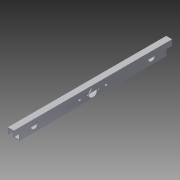
# Autodesk Inventor part: chassis side rail
Saved by Autodesk Inventor 2014 SP1 (Build 180222100, 222)
## iProperties
Created: 2014-01-04
Part Number: chassis side rail
Material: Aluminum 6061
Document SubType Name: Modeling
Designer: Arpan
Density: 2.71 g/cm^3
Appearance: Aluminum - Flat
Author: Arpan
Autodesk Inventor part; units mm, degrees
ref_plane "YZ Plane" through (0, 0, 0) normal (1, 0, 0) x (0, 1, 0)
ref_plane "XZ Plane" through (0, 0, 0) normal (0, 1, 0) x (-1, 0, 0)
ref_plane "XY Plane" through (0, 0, 0) normal (0, 0, 1) x (1, 0, 0)
sketch "Sketch1" plane through (0, 0, 0) normal (0, 0, 1) x (1, 0, 0)
  line L0 (0, 0) -> (-25.4, 0)
  line L1 (-25.4, 0) -> (-25.4, 50.8)
  line L2 (-25.4, 50.8) -> (0, 50.8)
  line L3 (0, 50.8) -> (0, 0)
  line L4 (-3.175, 47.625) -> (-22.225, 47.625)
  line L5 (-22.225, 47.625) -> (-22.225, 3.175)
  line L6 (-22.225, 3.175) -> (-3.175, 3.175)
  line L7 (-3.175, 3.175) -> (-3.175, 47.625)
  dimension "d0" = 25.4
  dimension "d1" = 50.8
  dimension "d2" = 3.175
  constraints: 16 end point, 4 parallel, 2 perpendicular, 1 horizontal, 3 other
  measures "d0" distance of L1.end L2.end
  measures "d1" distance of L2.end L0.start
  measures "d2" distance between parallel lines of L2 L4
extrude "Extrusion1" add sketch "Sketch1" along normal blind 685.8
sketch "Sketch2" plane through (0, 0, 0) normal (1, 0, 0) x (0, 0, -1)
  line L0 (0, 50.8) -> (0, 0) projected
  line L1 (-685.8, 0) -> (-685.8, 50.8) projected
  line L2 (0, 0) -> (-685.8, 0) projected
  line L3 (-685.8, 0) -> (-685.8, 25.4)
  line L4 (-685.8, 25.4) -> (-660.4, 25.4)
  line L5 (-660.4, 25.4) -> (-660.4, 0)
  line L6 (0, 25.4) -> (-25.4, 25.4)
  line L7 (-25.4, 25.4) -> (-25.4, 0)
  dimension "d5" = 25.4
  dimension "d6" = 25.4
  dimension "d7" = 25.4
  constraints: 10 end point, 4 perpendicular, 2 midpoint, 2 point on line
  measures "d5" distance of L1.start L3.end
  measures "d6" distance of L3.end L4.end
  measures "d7" distance of L6.start L6.end
extrude "Extrusion2" cut sketch "Sketch2" against normal blind 685.8
sketch "Sketch3" plane through (-25.4, 50.8, 0) normal (-1, 0, 0) x (0, 0, 1)
  line L0 (25.4, -50.8) -> (660.4, -50.8) projected
  line L1 (25.4, -50.8) -> (88.9, -50.8)
  line L2 (88.9, -50.8) -> (88.9, -23.8125)
  circle A0 centre (88.9, -23.8125) radius 14.2875
  line L3 (660.4, -50.8) -> (596.9, -50.8)
  line L4 (596.9, -50.8) -> (596.9, -23.8125)
  circle A1 centre (596.9, -23.8125) radius 14.2875
  line L5 (88.9, -50.8) -> (342.9, -50.8)
  line L6 (342.9, -50.8) -> (342.9, -23.8125)
  line L7 (342.9, -23.8125) -> (342.9, -26.9875)
  circle A2 centre (342.9, -26.9875) radius 19.05
  point P0 (0, -50.8)
  dimension "d10" = 63.5
  dimension "d11" = 26.9875
  dimension "d12" = 28.575
  dimension "d13" = 63.5
  dimension "d14" = 28.575
  dimension "d16" = 3.175
  dimension "d18" = 38.1
  constraints: 14 end point, 3 centre point, 3 coincident, 3 perpendicular, 3 point on line, 2 horizontal alignment, 1 midpoint
  measures "d10" distance of L0.start L1.end
  measures "d11" distance of L1.end L2.end
  measures "d12" diameter of A0
  measures "d13" distance of L0.end L3.end
  measures "d14" diameter of A1
  measures "d16" distance of L6.end L7.end
  measures "d18" diameter of A2
extrude "Extrusion3" cut sketch "Sketch3" against normal blind 685.8
sketch "Sketch4" plane through (-25.4, 50.8, 0) normal (-1, 0, 0) x (0, 0, 1)
  circle A0 centre (342.9, -26.9875) radius 19.05 projected
  line L0 (0, -25.4) -> (0, 0) projected
  line L1 (342.9, -26.9875) -> (319.0748, -26.9875)
  circle A1 centre (319.0748, -26.9875) radius 2.54
  line L2 (342.9, -26.9875) -> (366.7252, -26.9875)
  circle A2 centre (366.7252, -26.9875) radius 2.54
  line L3 (342.9, -26.9875) -> (285.75, -26.9875)
  line L4 (342.9, -26.9875) -> (400.05, -26.9875)
  circle A3 centre (285.75, -26.9875) radius 5.08
  circle A4 centre (400.05, -26.9875) radius 5.08
  point P0 (0, -50.8)
  dimension "d21" = 23.8252
  dimension "d22" = 5.08
  dimension "d23" = 23.8252
  dimension "d24" = 5.08
  dimension "d25" = 57.15
  dimension "d26" = 57.15
  dimension "d27" = 10.16
  constraints: 8 end point, 4 centre point, 4 coincident, 3 collinear, 1 perpendicular
  measures "d21" distance of L1.start L1.end
  measures "d22" diameter of A1
  measures "d23" distance of L1.start L2.end
  measures "d24" diameter of A2
  measures "d25" distance of L1.start L3.end
  measures "d26" distance of L1.start L4.end
  measures "d27" diameter of A3
extrude "Extrusion4" cut sketch "Sketch4" against normal blind 25.4 contours A1 L3 L1 | L1 L3 A1 | A2 L4 L2 | L2 L4 A2 | A3 | A4
body "Solid1"
